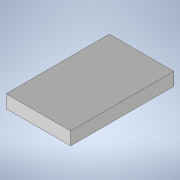
# Autodesk Inventor part: Peça2
Saved by Autodesk Inventor 2021 (Build 250183000, 183)
## iProperties
Created: 2022-02-01
Part Number: Peça2
Material: Genérico
Document SubType Name: Modeling
Designer: aluno
Density: 1 g/cm^3
Appearance: Padrão
Author: aluno
Autodesk Inventor part; units mm, degrees
ref_plane "YZ Plane" through (0, 0, 0) normal (1, 0, 0) x (0, 1, 0)
ref_plane "XZ Plane" through (0, 0, 0) normal (0, 1, 0) x (-1, 0, 0)
ref_plane "XY Plane" through (0, 0, 0) normal (0, 0, 1) x (1, 0, 0)
sketch "Esboço1" plane through (0, 0, 0) normal (0, 0, 1) x (1, 0, 0)
  line L0 (-80, -50) -> (80, -50)
  line L1 (80, -50) -> (80, 50)
  line L2 (80, 50) -> (-80, 50)
  line L3 (-80, 50) -> (-80, -50)
  line L4 (-80, -50) -> (80, 50) construction
  line L5 (80, -50) -> (-80, 50) construction
  point P0 (0, 0)
  dimension "d0" = 100
  dimension "d1" = 160
  constraints: 12 end point, 2 midpoint, 2 parallel, 1 horizontal, 1 perpendicular
  measures "d0" distance of L0.end L1.end
  measures "d1" distance of L0.start L0.end
extrude "Extrusão1" add sketch "Esboço1" along normal blind 20
